Autodesk Fusion 360 part; units mm, degrees
(part 2 of 2)
sketch "Sketch12" plane through (3, 0, 0) normal (1, 0, 0) x (0, 1, 0)
  line L0 (29.3, 0) -> (29.3, 33.5)
  line L1 (29.3, 33.5) -> (-3, 33.5)
  line L2 (-3, 33.5) -> (-3, 0)
  line L3 (-3, 0) -> (29.3, 0)
  spline S0 degree 3 poles (16.8231, 27.7956) (16.7769, 27.7883) (16.6969, 27.7776) (16.6456, 27.7708) knots 0 0 0 0 1 1 1 1
  spline S1 degree 3 poles (16.6456, 27.7708) (16.5335, 27.7568) (16.4265, 27.7404) (16.347, 27.7252) knots 0 0 0 0 1 1 1 1
  spline S2 degree 3 poles (16.347, 27.7252) (16.2124, 27.6987) (15.9471, 27.6266) (15.8192, 27.5815) knots 0 0 0 0 1 1 1 1
  spline S3 degree 3 poles (15.8192, 27.5815) (15.7702, 27.5641) (15.7088, 27.5427) (15.6823, 27.5331) knots 0 0 0 0 1 1 1 1
  spline S4 degree 3 poles (15.6823, 27.5331) (15.6558, 27.5241) (15.6271, 27.5134) (15.6175, 27.5089) knots 0 0 0 0 1 1 1 1
  spline S5 degree 3 poles (15.6175, 27.5089) (15.6085, 27.5049) (15.569, 27.4886) (15.5302, 27.4723) knots 0 0 0 0 1 1 1 1
  spline S6 degree 3 poles (15.5302, 27.4723) (15.4913, 27.4559) (15.4575, 27.4413) (15.4541, 27.4385) knots 0 0 0 0 1 1 1 1
  spline S7 degree 3 poles (15.4541, 27.4385) (15.4513, 27.4362) (15.4231, 27.4238) (15.3921, 27.4108) knots 0 0 0 0 1 1 1 1
  spline S8 degree 3 poles (15.3921, 27.4108) (15.3612, 27.3973) (15.3093, 27.3725) (15.2767, 27.3556) knots 0 0 0 0 1 1 1 1
  spline S9 degree 3 poles (15.2767, 27.3556) (15.244, 27.3382) (15.1888, 27.3094) (15.1544, 27.2914) knots 0 0 0 0 1 1 1 1
  spline S10 degree 3 poles (15.1544, 27.2914) (15.0609, 27.2435) (14.8051, 27.0869) (14.7499, 27.0447) knots 0 0 0 0 1 1 1 1
  spline S11 degree 3 poles (14.7499, 27.0447) (14.7375, 27.0351) (14.7082, 27.0142) (14.6851, 26.9979) knots 0 0 0 0 1 1 1 1
  spline S12 degree 3 poles (14.6851, 26.9979) (14.5792, 26.9247) (14.4277, 26.8069) (14.3105, 26.7066) knots 0 0 0 0 1 1 1 1
  spline S13 degree 3 poles (14.3105, 26.7066) (14.217, 26.6272) (14.1561, 26.5692) (14.0175, 26.43) knots 0 0 0 0 1 1 1 1
  spline S14 degree 3 poles (14.0175, 26.43) (13.8209, 26.2323) (13.817, 26.2283) (13.7522, 26.154) knots 0 0 0 0 1 1 1 1
  spline S15 degree 3 poles (13.7522, 26.154) (13.6406, 26.0272) (13.5837, 25.9562) (13.4299, 25.754) knots 0 0 0 0 1 1 1 1
  spline S16 degree 3 poles (13.4299, 25.754) (13.3916, 25.7038) (13.2761, 25.5326) (13.2006, 25.4148) knots 0 0 0 0 1 1 1 1
  spline S17 degree 3 poles (13.2006, 25.4148) (13.1145, 25.2796) (12.9691, 25.0013) (12.9077, 24.8526) knots 0 0 0 0 1 1 1 1
  spline S18 degree 3 poles (12.9077, 24.8526) (12.893, 24.8171) (12.875, 24.7754) (12.8683, 24.7596) knots 0 0 0 0 1 1 1 1
  spline S19 degree 3 poles (12.8683, 24.7596) (12.8491, 24.7157) (12.8316, 24.6706) (12.8294, 24.6571) knots 0 0 0 0 1 1 1 1
  spline S20 degree 3 poles (12.8294, 24.6571) (12.8277, 24.6503) (12.8153, 24.6137) (12.8018, 24.5754) knots 0 0 0 0 1 1 1 1
  spline S21 degree 3 poles (12.8018, 24.5754) (12.7809, 24.5168) (12.7623, 24.4611) (12.7297, 24.354) knots 0 0 0 0 1 1 1 1
  spline S22 degree 3 poles (12.7297, 24.354) (12.7269, 24.345) (12.7235, 24.3298) (12.7223, 24.3202) knots 0 0 0 0 1 1 1 1
  spline S23 degree 3 poles (12.7223, 24.3202) (12.7212, 24.3112) (12.71, 24.2616) (12.697, 24.2104) knots 0 0 0 0 1 1 1 1
  spline S24 degree 3 poles (12.697, 24.2104) (12.6514, 24.0239) (12.6215, 23.8419) (12.6147, 23.7061) knots 0 0 0 0 1 1 1 1
  spline S25 degree 3 poles (12.6147, 23.7061) (12.6136, 23.6785) (12.6097, 23.6177) (12.6069, 23.5709) knots 0 0 0 0 1 1 1 1
  spline S26 degree 3 poles (12.6069, 23.5709) (12.5995, 23.4645) (12.5995, 23.3062) (12.6063, 23.2076) knots 0 0 0 0 1 1 1 1
  spline S27 degree 3 poles (12.6063, 23.2076) (12.6097, 23.1659) (12.6131, 23.105) (12.6147, 23.0724) knots 0 0 0 0 1 1 1 1
  spline S28 degree 3 poles (12.6147, 23.0724) (12.6164, 23.0397) (12.6232, 22.9602) (12.63, 22.8955) knots 0 0 0 0 1 1 1 1
  line L4 (12.63, 22.8955) -> (12.6418, 22.7777)
  line L5 (12.6418, 22.7777) -> (12.7466, 22.7817)
  spline S29 degree 3 poles (12.7466, 22.7817) (12.9922, 22.7907) (13.2373, 22.8177) (13.4654, 22.8617) knots 0 0 0 0 1 1 1 1
  spline S30 degree 3 poles (13.4654, 22.8617) (13.6063, 22.8887) (13.8863, 22.9698) (14.0271, 23.0245) knots 0 0 0 0 1 1 1 1
  spline S31 degree 3 poles (14.0271, 23.0245) (14.0879, 23.0476) (14.1392, 23.0667) (14.1415, 23.0667) knots 0 0 0 0 1 1 1 1
  spline S32 degree 3 poles (14.1415, 23.0667) (14.1437, 23.0667) (14.1589, 23.0729) (14.1747, 23.0802) knots 0 0 0 0 1 1 1 1
  spline S33 degree 3 poles (14.1747, 23.0802) (14.1905, 23.0876) (14.2277, 23.1045) (14.257, 23.1174) knots 0 0 0 0 1 1 1 1
  spline S34 degree 3 poles (14.257, 23.1174) (14.3122, 23.1417) (14.3206, 23.1456) (14.4485, 23.2104) knots 0 0 0 0 1 1 1 1
  spline S35 degree 3 poles (14.4485, 23.2104) (14.5662, 23.2695) (14.8367, 23.4278) (14.8485, 23.4442) knots 0 0 0 0 1 1 1 1
  spline S36 degree 3 poles (14.8485, 23.4442) (14.8502, 23.4464) (14.8795, 23.4673) (14.9133, 23.4904) knots 0 0 0 0 1 1 1 1
  spline S37 degree 3 poles (14.9133, 23.4904) (14.9967, 23.5473) (15.0958, 23.62) (15.1809, 23.6887) knots 0 0 0 0 1 1 1 1
  spline S38 degree 3 poles (15.1809, 23.6887) (15.2474, 23.7422) (15.2676, 23.7597) (15.3747, 23.8571) knots 0 0 0 0 1 1 1 1
  spline S39 degree 3 poles (15.3747, 23.8571) (15.533, 24.0008) (15.7921, 24.2695) (15.911, 24.4132) knots 0 0 0 0 1 1 1 1
  spline S40 degree 3 poles (15.911, 24.4132) (15.9589, 24.4712) (16.0958, 24.652) (16.1414, 24.718) knots 0 0 0 0 1 1 1 1
  spline S41 degree 3 poles (16.1414, 24.718) (16.1572, 24.7405) (16.173, 24.7619) (16.1769, 24.7658) knots 0 0 0 0 1 1 1 1
  spline S42 degree 3 poles (16.1769, 24.7658) (16.1876, 24.7771) (16.3093, 24.9698) (16.3335, 25.0137) knots 0 0 0 0 1 1 1 1
  spline S43 degree 3 poles (16.3335, 25.0137) (16.3448, 25.0351) (16.36, 25.0605) (16.3673, 25.0706) knots 0 0 0 0 1 1 1 1
  spline S44 degree 3 poles (16.3673, 25.0706) (16.3825, 25.0909) (16.5386, 25.3895) (16.5386, 25.3979) knots 0 0 0 0 1 1 1 1
  spline S45 degree 3 poles (16.5386, 25.3979) (16.5386, 25.4008) (16.5516, 25.4312) (16.5673, 25.4644) knots 0 0 0 0 1 1 1 1
  spline S46 degree 3 poles (16.5673, 25.4644) (16.6011, 25.5371) (16.6456, 25.6436) (16.649, 25.6605) knots 0 0 0 0 1 1 1 1
  spline S47 degree 3 poles (16.649, 25.6605) (16.6501, 25.6672) (16.6535, 25.6774) (16.6569, 25.6836) knots 0 0 0 0 1 1 1 1
  spline S48 degree 3 poles (16.6569, 25.6836) (16.6761, 25.7213) (16.7448, 25.9224) (16.7504, 25.9568) knots 0 0 0 0 1 1 1 1
  spline S49 degree 3 poles (16.7504, 25.9568) (16.7515, 25.9647) (16.7566, 25.981) (16.7611, 25.9934) knots 0 0 0 0 1 1 1 1
  spline S50 degree 3 poles (16.7611, 25.9934) (16.7752, 26.0329) (16.8361, 26.2706) (16.8484, 26.3331) knots 0 0 0 0 1 1 1 1
  spline S51 degree 3 poles (16.8484, 26.3331) (16.8817, 26.5083) (16.9087, 26.7061) (16.9256, 26.8892) knots 0 0 0 0 1 1 1 1
  spline S52 degree 3 poles (16.9256, 26.8892) (16.942, 27.0728) (16.938, 27.5494) (16.9183, 27.7725) knots 0 0 0 0 1 1 1 1
  spline S53 degree 3 poles (16.9183, 27.7725) (16.916, 27.7934) (16.9132, 27.8097) (16.911, 27.8097) knots 0 0 0 0 1 1 1 1
  spline S54 degree 3 poles (16.911, 27.8097) (16.9093, 27.8091) (16.8699, 27.8029) (16.8231, 27.7956) knots 0 0 0 0 1 1 1 1
  spline S55 degree 3 poles (9.1782, 23.0498) (8.8909, 23.0335) (8.6036, 23.0002) (8.3163, 22.9507) knots 0 0 0 0 1 1 1 1
  spline S56 degree 3 poles (8.3163, 22.9507) (8.1613, 22.9236) (7.8334, 22.8414) (7.674, 22.7901) knots 0 0 0 0 1 1 1 1
  spline S57 degree 3 poles (7.674, 22.7901) (7.5208, 22.7405) (7.4537, 22.718) (7.4318, 22.709) knots 0 0 0 0 1 1 1 1
  spline S58 degree 3 poles (7.4318, 22.709) (7.4228, 22.7045) (7.3591, 22.6797) (7.2915, 22.6526) knots 0 0 0 0 1 1 1 1
  spline S59 degree 3 poles (7.2915, 22.6526) (7.2239, 22.6262) (7.145, 22.5929) (7.1168, 22.5794) knots 0 0 0 0 1 1 1 1
  spline S60 degree 3 poles (7.1168, 22.5794) (7.0887, 22.5659) (7.0329, 22.54) (6.9923, 22.5214) knots 0 0 0 0 1 1 1 1
  spline S61 degree 3 poles (6.9923, 22.5214) (6.9523, 22.5034) (6.8966, 22.4752) (6.8684, 22.4589) knots 0 0 0 0 1 1 1 1
  spline S62 degree 3 poles (6.8684, 22.4589) (6.8408, 22.4431) (6.816, 22.4301) (6.8138, 22.4301) knots 0 0 0 0 1 1 1 1
  spline S63 degree 3 poles (6.8138, 22.4301) (6.7985, 22.4301) (6.469, 22.2335) (6.3783, 22.1698) knots 0 0 0 0 1 1 1 1
  spline S64 degree 3 poles (6.3783, 22.1698) (6.2059, 22.0498) (6.0465, 21.9287) (5.9276, 21.8284) knots 0 0 0 0 1 1 1 1
  spline S65 degree 3 poles (5.9276, 21.8284) (5.7873, 21.7096) (5.4853, 21.4104) (5.3608, 21.2662) knots 0 0 0 0 1 1 1 1
  spline S66 degree 3 poles (5.3608, 21.2662) (5.2566, 21.1462) (5.1738, 21.042) (5.0769, 20.909) knots 0 0 0 0 1 1 1 1
  spline S67 degree 3 poles (5.0769, 20.909) (5.0459, 20.8673) (5.0177, 20.8296) (5.0138, 20.8257) knots 0 0 0 0 1 1 1 1
  spline S68 degree 3 poles (5.0138, 20.8257) (5.0037, 20.8155) (4.8876, 20.6397) (4.8454, 20.571) knots 0 0 0 0 1 1 1 1
  spline S69 degree 3 poles (4.8454, 20.571) (4.8273, 20.5417) (4.811, 20.5164) (4.8093, 20.5147) knots 0 0 0 0 1 1 1 1
  spline S70 degree 3 poles (4.8093, 20.5147) (4.7941, 20.5028) (4.6409, 20.224) (4.5687, 20.0775) knots 0 0 0 0 1 1 1 1
  spline S71 degree 3 poles (4.5687, 20.0775) (4.4865, 19.9113) (4.46, 19.8538) (4.4149, 19.7457) knots 0 0 0 0 1 1 1 1
  spline S72 degree 3 poles (4.4149, 19.7457) (4.3547, 19.6009) (4.3406, 19.566) (4.3383, 19.5541) knots 0 0 0 0 1 1 1 1
  spline S73 degree 3 poles (4.3383, 19.5541) (4.3372, 19.5479) (4.3299, 19.5265) (4.322, 19.5062) knots 0 0 0 0 1 1 1 1
  spline S74 degree 3 poles (4.322, 19.5062) (4.3006, 19.4539) (4.2403, 19.2854) (4.2386, 19.2753) knots 0 0 0 0 1 1 1 1
  spline S75 degree 3 poles (4.2386, 19.2753) (4.2375, 19.2708) (4.2352, 19.2634) (4.233, 19.2601) knots 0 0 0 0 1 1 1 1
  spline S76 degree 3 poles (4.233, 19.2601) (4.2302, 19.2561) (4.2296, 19.2527) (4.2307, 19.2527) knots 0 0 0 0 1 1 1 1
  spline S77 degree 3 poles (4.2307, 19.2527) (4.2324, 19.2527) (4.2262, 19.2291) (4.2166, 19.2009) knots 0 0 0 0 1 1 1 1
  spline S78 degree 3 poles (4.2166, 19.2009) (4.1755, 19.0708) (4.1366, 18.9384) (4.1316, 18.9091) knots 0 0 0 0 1 1 1 1
  spline S79 degree 3 poles (4.1316, 18.9091) (4.1299, 18.9012) (4.1186, 18.8539) (4.1057, 18.8037) knots 0 0 0 0 1 1 1 1
  spline S80 degree 3 poles (4.1057, 18.8037) (4.0679, 18.6539) (4.0279, 18.4708) (4.0228, 18.428) knots 0 0 0 0 1 1 1 1
  spline S81 degree 3 poles (4.0228, 18.428) (4.0217, 18.4156) (4.0166, 18.384) (4.0121, 18.3575) knots 0 0 0 0 1 1 1 1
  spline S82 degree 3 poles (4.0121, 18.3575) (3.9631, 18.0871) (3.9231, 17.7852) (3.9169, 17.6443) knots 0 0 0 0 1 1 1 1
  spline S83 degree 3 poles (3.9169, 17.6443) (3.9152, 17.6105) (3.9102, 17.5294) (3.9057, 17.464) knots 0 0 0 0 1 1 1 1
  spline S84 degree 3 poles (3.9057, 17.464) (3.8893, 17.2364) (3.8837, 17.0173) (3.8871, 16.7204) knots 0 0 0 0 1 1 1 1
  spline S85 degree 3 poles (3.8871, 16.7204) (3.8904, 16.4393) (3.8938, 16.3463) (3.9107, 16.0951) knots 0 0 0 0 1 1 1 1
  spline S86 degree 3 poles (3.9107, 16.0951) (3.9147, 16.0269) (3.9186, 15.957) (3.9186, 15.9401) knots 0 0 0 0 1 1 1 1
  spline S87 degree 3 poles (3.9186, 15.9401) (3.9192, 15.8522) (3.9721, 15.4027) (4.0093, 15.1655) knots 0 0 0 0 1 1 1 1
  spline S88 degree 3 poles (4.0093, 15.1655) (4.0149, 15.1283) (4.0217, 15.0804) (4.0234, 15.0596) knots 0 0 0 0 1 1 1 1
  spline S89 degree 3 poles (4.0234, 15.0596) (4.0262, 15.0264) (4.0437, 14.9244) (4.0741, 14.7627) knots 0 0 0 0 1 1 1 1
  spline S90 degree 3 poles (4.0741, 14.7627) (4.0792, 14.7362) (4.0933, 14.6669) (4.1057, 14.6078) knots 0 0 0 0 1 1 1 1
  spline S91 degree 3 poles (4.1057, 14.6078) (4.1175, 14.5492) (4.1287, 14.49) (4.1299, 14.4776) knots 0 0 0 0 1 1 1 1
  spline S92 degree 3 poles (4.1299, 14.4776) (4.1327, 14.45) (4.1513, 14.3672) (4.1935, 14.1965) knots 0 0 0 0 1 1 1 1
  spline S93 degree 3 poles (4.1935, 14.1965) (4.2104, 14.1283) (4.2279, 14.0551) (4.2318, 14.0331) knots 0 0 0 0 1 1 1 1
  spline S94 degree 3 poles (4.2318, 14.0331) (4.2425, 13.9791) (4.2831, 13.8275) (4.3299, 13.6686) knots 0 0 0 0 1 1 1 1
  spline S95 degree 3 poles (4.3299, 13.6686) (4.3361, 13.6472) (4.3394, 13.6303) (4.3378, 13.6303) knots 0 0 0 0 1 1 1 1
  spline S96 degree 3 poles (4.3378, 13.6303) (4.3361, 13.6303) (4.3378, 13.627) (4.3411, 13.623) knots 0 0 0 0 1 1 1 1
  spline S97 degree 3 poles (4.3411, 13.623) (4.3445, 13.6185) (4.3462, 13.614) (4.3445, 13.6123) knots 0 0 0 0 1 1 1 1
  spline S98 degree 3 poles (4.3445, 13.6123) (4.3417, 13.6095) (4.3547, 13.5655) (4.4132, 13.3824) knots 0 0 0 0 1 1 1 1
  spline S99 degree 3 poles (4.4132, 13.3824) (4.4307, 13.3284) (4.4454, 13.2788) (4.4465, 13.2726) knots 0 0 0 0 1 1 1 1
  spline S100 degree 3 poles (4.4465, 13.2726) (4.4471, 13.2664) (4.4707, 13.1948) (4.4989, 13.1132) knots 0 0 0 0 1 1 1 1
  spline S101 degree 3 poles (4.4989, 13.1132) (4.5271, 13.0315) (4.5513, 12.9594) (4.5524, 12.9526) knots 0 0 0 0 1 1 1 1
  spline S102 degree 3 poles (4.5524, 12.9526) (4.5552, 12.9402) (4.5992, 12.818) (4.6369, 12.7182) knots 0 0 0 0 1 1 1 1
  spline S103 degree 3 poles (4.6369, 12.7182) (4.6482, 12.6895) (4.6572, 12.663) (4.6572, 12.6596) knots 0 0 0 0 1 1 1 1
  spline S104 degree 3 poles (4.6572, 12.6596) (4.6572, 12.6568) (4.6825, 12.5904) (4.713, 12.5126) knots 0 0 0 0 1 1 1 1
  spline S105 degree 3 poles (4.713, 12.5126) (4.7439, 12.4349) (4.7777, 12.3487) (4.789, 12.3205) knots 0 0 0 0 1 1 1 1
  spline S106 degree 3 poles (4.789, 12.3205) (4.7997, 12.2929) (4.8228, 12.2371) (4.8403, 12.1966) knots 0 0 0 0 1 1 1 1
  spline S107 degree 3 poles (4.8403, 12.1966) (4.8577, 12.1566) (4.873, 12.1188) (4.8741, 12.1137) knots 0 0 0 0 1 1 1 1
  spline S108 degree 3 poles (4.8741, 12.1137) (4.8752, 12.1087) (4.8927, 12.0681) (4.9124, 12.0236) knots 0 0 0 0 1 1 1 1
  spline S109 degree 3 poles (4.9124, 12.0236) (4.9321, 11.9791) (4.967, 11.9014) (4.9896, 11.8501) knots 0 0 0 0 1 1 1 1
  spline S110 degree 3 poles (4.9896, 11.8501) (5.0121, 11.7988) (5.0414, 11.7346) (5.0555, 11.7064) knots 0 0 0 0 1 1 1 1
  spline S111 degree 3 poles (5.0555, 11.7064) (5.0696, 11.6788) (5.082, 11.6512) (5.0831, 11.6456) knots 0 0 0 0 1 1 1 1
  spline S112 degree 3 poles (5.0831, 11.6456) (5.0876, 11.6197) (5.4177, 10.9622) (5.478, 10.8586) knots 0 0 0 0 1 1 1 1
  spline S113 degree 3 poles (5.478, 10.8586) (5.4876, 10.8417) (5.5056, 10.8084) (5.5174, 10.7853) knots 0 0 0 0 1 1 1 1
  spline S114 degree 3 poles (5.5174, 10.7853) (5.558, 10.7087) (5.6222, 10.591) (5.6318, 10.5769) knots 0 0 0 0 1 1 1 1
  spline S115 degree 3 poles (5.6318, 10.5769) (5.6369, 10.569) (5.6611, 10.5273) (5.6853, 10.4839) knots 0 0 0 0 1 1 1 1
  spline S116 degree 3 poles (5.6853, 10.4839) (5.7096, 10.4405) (5.7372, 10.3921) (5.7467, 10.3763) knots 0 0 0 0 1 1 1 1
  spline S117 degree 3 poles (5.7467, 10.3763) (5.7563, 10.36) (5.7783, 10.3234) (5.7958, 10.2946) knots 0 0 0 0 1 1 1 1
  spline S118 degree 3 poles (5.7958, 10.2946) (5.8132, 10.2653) (5.838, 10.2225) (5.8515, 10.1994) knots 0 0 0 0 1 1 1 1
  spline S119 degree 3 poles (5.8515, 10.1994) (5.865, 10.1763) (5.8881, 10.1386) (5.9034, 10.116) knots 0 0 0 0 1 1 1 1
  spline S120 degree 3 poles (5.9034, 10.116) (5.918, 10.0935) (5.9304, 10.0744) (5.9304, 10.0727) knots 0 0 0 0 1 1 1 1
  spline S121 degree 3 poles (5.9304, 10.0727) (5.9304, 10.0715) (5.9546, 10.0315) (5.9839, 9.9848) knots 0 0 0 0 1 1 1 1
  spline S122 degree 3 poles (5.9839, 9.9848) (6.0132, 9.938) (6.0374, 9.8986) (6.0374, 9.8975) knots 0 0 0 0 1 1 1 1
  spline S123 degree 3 poles (6.0374, 9.8975) (6.0374, 9.8958) (6.0797, 9.8315) (6.1129, 9.7825) knots 0 0 0 0 1 1 1 1
  spline S124 degree 3 poles (6.1129, 9.7825) (6.1203, 9.7718) (6.1597, 9.711) (6.2014, 9.6473) knots 0 0 0 0 1 1 1 1
  spline S125 degree 3 poles (6.2014, 9.6473) (6.2425, 9.5837) (6.2938, 9.5076) (6.3152, 9.4783) knots 0 0 0 0 1 1 1 1
  spline S126 degree 3 poles (6.3152, 9.4783) (6.336, 9.449) (6.3884, 9.3752) (6.4312, 9.3149) knots 0 0 0 0 1 1 1 1
  spline S127 degree 3 poles (6.4312, 9.3149) (6.5095, 9.2034) (6.5811, 9.1071) (6.6374, 9.0361) knots 0 0 0 0 1 1 1 1
  spline S128 degree 3 poles (6.6374, 9.0361) (6.6549, 9.0147) (6.6949, 8.964) (6.7264, 8.9234) knots 0 0 0 0 1 1 1 1
  spline S129 degree 3 poles (6.7264, 8.9234) (6.8307, 8.7899) (6.9907, 8.5995) (7.0599, 8.5262) knots 0 0 0 0 1 1 1 1
  spline S130 degree 3 poles (7.0599, 8.5262) (7.3157, 8.2569) (7.4656, 8.111) (7.6137, 7.9865) knots 0 0 0 0 1 1 1 1
  spline S131 degree 3 poles (7.6137, 7.9865) (7.8205, 7.813) (8.0357, 7.6603) (8.2194, 7.5567) knots 0 0 0 0 1 1 1 1
  spline S132 degree 3 poles (8.2194, 7.5567) (8.2436, 7.5432) (8.2802, 7.5223) (8.301, 7.5105) knots 0 0 0 0 1 1 1 1
  spline S133 degree 3 poles (8.301, 7.5105) (8.3219, 7.4981) (8.3692, 7.4744) (8.4064, 7.4575) knots 0 0 0 0 1 1 1 1
  spline S134 degree 3 poles (8.4064, 7.4575) (8.4436, 7.4406) (8.4768, 7.4243) (8.4796, 7.4215) knots 0 0 0 0 1 1 1 1
  spline S135 degree 3 poles (8.4796, 7.4215) (8.4892, 7.4141) (8.5771, 7.377) (8.6148, 7.3646) knots 0 0 0 0 1 1 1 1
  spline S136 degree 3 poles (8.6148, 7.3646) (8.6334, 7.3584) (8.6565, 7.3499) (8.6655, 7.3454) knots 0 0 0 0 1 1 1 1
  spline S137 degree 3 poles (8.6655, 7.3454) (8.7129, 7.324) (8.8903, 7.2671) (8.9371, 7.2587) knots 0 0 0 0 1 1 1 1
  spline S138 degree 3 poles (8.9371, 7.2587) (8.9517, 7.2564) (8.9991, 7.2463) (9.0413, 7.2372) knots 0 0 0 0 1 1 1 1
  spline S139 degree 3 poles (9.0413, 7.2372) (9.319, 7.1753) (9.6148, 7.1691) (9.9585, 7.217) knots 0 0 0 0 1 1 1 1
  spline S140 degree 3 poles (9.9585, 7.217) (10.0396, 7.2282) (10.19, 7.2558) (10.2683, 7.2733) knots 0 0 0 0 1 1 1 1
  spline S141 degree 3 poles (10.2683, 7.2733) (10.3641, 7.2953) (10.6351, 7.3786) (10.6897, 7.4029) knots 0 0 0 0 1 1 1 1
  spline S142 degree 3 poles (10.6897, 7.4029) (10.7072, 7.4108) (10.7928, 7.4463) (10.8796, 7.4823) knots 0 0 0 0 1 1 1 1
  spline S143 degree 3 poles (10.8796, 7.4823) (10.9663, 7.5178) (11.0401, 7.5488) (11.043, 7.551) knots 0 0 0 0 1 1 1 1
  spline S144 degree 3 poles (11.043, 7.551) (11.0463, 7.5533) (11.0638, 7.5612) (11.0824, 7.5679) knots 0 0 0 0 1 1 1 1
  spline S145 degree 3 poles (11.0824, 7.5679) (11.101, 7.5753) (11.1477, 7.5939) (11.1866, 7.6091) knots 0 0 0 0 1 1 1 1
  spline S146 degree 3 poles (11.1866, 7.6091) (11.2255, 7.6248) (11.3105, 7.6558) (11.3753, 7.6784) knots 0 0 0 0 1 1 1 1
  spline S147 degree 3 poles (11.3753, 7.6784) (11.4407, 7.7009) (11.5117, 7.7262) (11.5331, 7.7341) knots 0 0 0 0 1 1 1 1
  spline S148 degree 3 poles (11.5331, 7.7341) (11.6007, 7.76) (11.6841, 7.7893) (11.7105, 7.7967) knots 0 0 0 0 1 1 1 1
  spline S149 degree 3 poles (11.7105, 7.7967) (11.7246, 7.8006) (11.7872, 7.8203) (11.8497, 7.8406) knots 0 0 0 0 1 1 1 1
  spline S150 degree 3 poles (11.8497, 7.8406) (11.9719, 7.8806) (12.3026, 7.9646) (12.426, 7.9876) knots 0 0 0 0 1 1 1 1
  spline S151 degree 3 poles (12.426, 7.9876) (12.5026, 8.0017) (12.7184, 8.031) (12.8232, 8.0417) knots 0 0 0 0 1 1 1 1
  spline S152 degree 3 poles (12.8232, 8.0417) (13.0784, 8.0676) (13.4418, 8.0564) (13.7499, 8.0136) knots 0 0 0 0 1 1 1 1
  spline S153 degree 3 poles (13.7499, 8.0136) (13.7916, 8.0079) (13.8401, 8.0017) (13.857, 7.9995) knots 0 0 0 0 1 1 1 1
  spline S154 degree 3 poles (13.857, 7.9995) (13.9088, 7.9938) (14.0857, 7.9527) (14.1753, 7.9262) knots 0 0 0 0 1 1 1 1
  spline S155 degree 3 poles (14.1753, 7.9262) (14.222, 7.9122) (14.2727, 7.8969) (14.2891, 7.8924) knots 0 0 0 0 1 1 1 1
  spline S156 degree 3 poles (14.2891, 7.8924) (14.3054, 7.8879) (14.3612, 7.8677) (14.413, 7.8468) knots 0 0 0 0 1 1 1 1
  spline S157 degree 3 poles (14.413, 7.8468) (14.4648, 7.8265) (14.5257, 7.804) (14.5471, 7.7967) knots 0 0 0 0 1 1 1 1
  spline S158 degree 3 poles (14.5471, 7.7967) (14.5691, 7.7893) (14.626, 7.7679) (14.6738, 7.7488) knots 0 0 0 0 1 1 1 1
  spline S159 degree 3 poles (14.6738, 7.7488) (14.7217, 7.7302) (14.7792, 7.7082) (14.8006, 7.7003) knots 0 0 0 0 1 1 1 1
  spline S160 degree 3 poles (14.8006, 7.7003) (14.8913, 7.6671) (14.92, 7.6564) (14.9443, 7.6457) knots 0 0 0 0 1 1 1 1
  spline S161 degree 3 poles (14.9443, 7.6457) (14.9809, 7.6293) (15.2682, 7.5212) (15.3443, 7.4947) knots 0 0 0 0 1 1 1 1
  spline S162 degree 3 poles (15.3443, 7.4947) (15.5043, 7.4401) (15.6276, 7.3989) (15.6795, 7.3837) knots 0 0 0 0 1 1 1 1
  spline S163 degree 3 poles (15.6795, 7.3837) (16.0118, 7.2846) (16.2676, 7.2288) (16.5442, 7.1956) knots 0 0 0 0 1 1 1 1
  spline S164 degree 3 poles (16.5442, 7.1956) (16.6349, 7.1843) (16.8907, 7.1865) (16.9775, 7.1984) knots 0 0 0 0 1 1 1 1
  spline S165 degree 3 poles (16.9775, 7.1984) (17.1634, 7.2249) (17.3651, 7.2789) (17.5115, 7.3409) knots 0 0 0 0 1 1 1 1
  spline S166 degree 3 poles (17.5115, 7.3409) (17.5436, 7.3544) (17.5729, 7.3657) (17.5769, 7.3657) knots 0 0 0 0 1 1 1 1
  spline S167 degree 3 poles (17.5769, 7.3657) (17.5848, 7.3657) (17.8405, 7.493) (17.8879, 7.5206) knots 0 0 0 0 1 1 1 1
  spline S168 degree 3 poles (17.8879, 7.5206) (17.9036, 7.5296) (17.9301, 7.5465) (17.9476, 7.5584) knots 0 0 0 0 1 1 1 1
  spline S169 degree 3 poles (17.9476, 7.5584) (17.965, 7.5702) (17.9814, 7.5798) (17.9831, 7.5798) knots 0 0 0 0 1 1 1 1
  spline S170 degree 3 poles (17.9831, 7.5798) (17.9898, 7.5798) (18.1538, 7.6862) (18.205, 7.7234) knots 0 0 0 0 1 1 1 1
  spline S171 degree 3 poles (18.205, 7.7234) (18.2991, 7.7916) (18.3115, 7.8012) (18.3746, 7.8491) knots 0 0 0 0 1 1 1 1
  spline S172 degree 3 poles (18.3746, 7.8491) (18.7661, 8.1482) (19.1706, 8.5471) (19.5813, 9.0389) knots 0 0 0 0 1 1 1 1
  spline S173 degree 3 poles (19.5813, 9.0389) (19.7892, 9.2885) (19.9058, 9.4372) (20.0416, 9.6259) knots 0 0 0 0 1 1 1 1
  spline S174 degree 3 poles (20.0416, 9.6259) (20.0698, 9.6648) (20.0979, 9.7031) (20.1047, 9.7104) knots 0 0 0 0 1 1 1 1
  spline S175 degree 3 poles (20.1047, 9.7104) (20.1182, 9.7268) (20.1492, 9.7707) (20.2427, 9.9093) knots 0 0 0 0 1 1 1 1
  spline S176 degree 3 poles (20.2427, 9.9093) (20.2805, 9.9651) (20.3216, 10.0248) (20.3346, 10.0417) knots 0 0 0 0 1 1 1 1
  spline S177 degree 3 poles (20.3346, 10.0417) (20.3475, 10.0586) (20.3582, 10.0744) (20.3582, 10.0766) knots 0 0 0 0 1 1 1 1
  spline S178 degree 3 poles (20.3582, 10.0766) (20.3582, 10.0789) (20.3819, 10.1166) (20.4106, 10.1611) knots 0 0 0 0 1 1 1 1
  spline S179 degree 3 poles (20.4106, 10.1611) (20.4399, 10.2056) (20.4647, 10.2445) (20.4658, 10.2484) knots 0 0 0 0 1 1 1 1
  spline S180 degree 3 poles (20.4658, 10.2484) (20.467, 10.2518) (20.4889, 10.2873) (20.5148, 10.3273) knots 0 0 0 0 1 1 1 1
  spline S181 degree 3 poles (20.5148, 10.3273) (20.5627, 10.4005) (20.6726, 10.5842) (20.6782, 10.5994) knots 0 0 0 0 1 1 1 1
  spline S182 degree 3 poles (20.6782, 10.5994) (20.6799, 10.6039) (20.6867, 10.6158) (20.6934, 10.6248) knots 0 0 0 0 1 1 1 1
  spline S183 degree 3 poles (20.6934, 10.6248) (20.7092, 10.6467) (20.7509, 10.72) (20.7869, 10.7893) knots 0 0 0 0 1 1 1 1
  spline S184 degree 3 poles (20.7869, 10.7893) (20.8033, 10.8197) (20.8213, 10.8518) (20.8275, 10.8603) knots 0 0 0 0 1 1 1 1
  spline S185 degree 3 poles (20.8275, 10.8603) (20.8602, 10.9076) (21.2061, 11.5943) (21.2117, 11.6242) knots 0 0 0 0 1 1 1 1
  spline S186 degree 3 poles (21.2117, 11.6242) (21.2128, 11.6293) (21.223, 11.6523) (21.2343, 11.6754) knots 0 0 0 0 1 1 1 1
  spline S187 degree 3 poles (21.2343, 11.6754) (21.2641, 11.7363) (21.3041, 11.8259) (21.3159, 11.8585) knots 0 0 0 0 1 1 1 1
  spline S188 degree 3 poles (21.3159, 11.8585) (21.3255, 11.8839) (21.3458, 11.9307) (21.401, 12.054) knots 0 0 0 0 1 1 1 1
  spline S189 degree 3 poles (21.401, 12.054) (21.41, 12.0743) (21.419, 12.0963) (21.4202, 12.1019) knots 0 0 0 0 1 1 1 1
  spline S190 degree 3 poles (21.4202, 12.1019) (21.4213, 12.1076) (21.4354, 12.1436) (21.4512, 12.1825) knots 0 0 0 0 1 1 1 1
  spline S191 degree 3 poles (21.4512, 12.1825) (21.5002, 12.3008) (21.5289, 12.374) (21.5266, 12.374) knots 0 0 0 0 1 1 1 1
  spline S192 degree 3 poles (21.5266, 12.374) (21.5244, 12.374) (21.543, 12.4247) (21.5526, 12.4444) knots 0 0 0 0 1 1 1 1
  spline S193 degree 3 poles (21.5526, 12.4444) (21.5559, 12.4506) (21.5689, 12.4839) (21.5813, 12.5177) knots 0 0 0 0 1 1 1 1
  spline S194 degree 3 poles (21.5813, 12.5177) (21.5942, 12.552) (21.6117, 12.5982) (21.6202, 12.6208) knots 0 0 0 0 1 1 1 1
  spline S195 degree 3 poles (21.6202, 12.6208) (21.6292, 12.6427) (21.6348, 12.6613) (21.6337, 12.6613) knots 0 0 0 0 1 1 1 1
  spline S196 degree 3 poles (21.6337, 12.6613) (21.6326, 12.6613) (21.6393, 12.6833) (21.6489, 12.7098) knots 0 0 0 0 1 1 1 1
  spline S197 degree 3 poles (21.6489, 12.7098) (21.6585, 12.7363) (21.6652, 12.7594) (21.6641, 12.7599) knots 0 0 0 0 1 1 1 1
  spline S198 degree 3 poles (21.6641, 12.7599) (21.663, 12.7611) (21.6455, 12.7695) (21.6252, 12.7785) knots 0 0 0 0 1 1 1 1
  spline S199 degree 3 poles (21.6252, 12.7785) (21.605, 12.7875) (21.5548, 12.8146) (21.5142, 12.8382) knots 0 0 0 0 1 1 1 1
  spline S200 degree 3 poles (21.5142, 12.8382) (21.4731, 12.8619) (21.4382, 12.8811) (21.4359, 12.8811) knots 0 0 0 0 1 1 1 1
  spline S201 degree 3 poles (21.4359, 12.8811) (21.4309, 12.8811) (21.3345, 12.9363) (21.2923, 12.9639) knots 0 0 0 0 1 1 1 1
  spline S202 degree 3 poles (21.2923, 12.9639) (21.2714, 12.9774) (21.2534, 12.9881) (21.2512, 12.9881) knots 0 0 0 0 1 1 1 1
  spline S203 degree 3 poles (21.2512, 12.9881) (21.2438, 12.9881) (21.0607, 13.1036) (20.9447, 13.1808) knots 0 0 0 0 1 1 1 1
  spline S204 degree 3 poles (20.9447, 13.1808) (20.7819, 13.2901) (20.7188, 13.3346) (20.6399, 13.3965) knots 0 0 0 0 1 1 1 1
  spline S205 degree 3 poles (20.6399, 13.3965) (20.6202, 13.4123) (20.5746, 13.4472) (20.5391, 13.4754) knots 0 0 0 0 1 1 1 1
  spline S206 degree 3 poles (20.5391, 13.4754) (20.3199, 13.645) (20.0692, 13.8765) (19.8929, 14.0726) knots 0 0 0 0 1 1 1 1
  spline S207 degree 3 poles (19.8929, 14.0726) (19.716, 14.2698) (19.5211, 14.5312) (19.3971, 14.7368) knots 0 0 0 0 1 1 1 1
  spline S208 degree 3 poles (19.3971, 14.7368) (19.3791, 14.7672) (19.3566, 14.8038) (19.3475, 14.8185) knots 0 0 0 0 1 1 1 1
  spline S209 degree 3 poles (19.3475, 14.8185) (19.3385, 14.8326) (19.3188, 14.8686) (19.3036, 14.8979) knots 0 0 0 0 1 1 1 1
  spline S210 degree 3 poles (19.3036, 14.8979) (19.2878, 14.9272) (19.2591, 14.9818) (19.2399, 15.019) knots 0 0 0 0 1 1 1 1
  spline S211 degree 3 poles (19.2399, 15.019) (19.2202, 15.0562) (19.1949, 15.108) (19.1836, 15.134) knots 0 0 0 0 1 1 1 1
  spline S212 degree 3 poles (19.1836, 15.134) (19.1723, 15.1604) (19.1571, 15.1948) (19.1492, 15.21) knots 0 0 0 0 1 1 1 1
  spline S213 degree 3 poles (19.1492, 15.21) (19.1301, 15.2478) (19.0935, 15.3362) (19.0884, 15.3565) knots 0 0 0 0 1 1 1 1
  spline S214 degree 3 poles (19.0884, 15.3565) (19.0861, 15.3649) (19.0794, 15.383) (19.0737, 15.3959) knots 0 0 0 0 1 1 1 1
  spline S215 degree 3 poles (19.0737, 15.3959) (19.0506, 15.4444) (18.9859, 15.6263) (18.9814, 15.6545) knots 0 0 0 0 1 1 1 1
  spline S216 degree 3 poles (18.9814, 15.6545) (18.9797, 15.6641) (18.9735, 15.6877) (18.9673, 15.7063) knots 0 0 0 0 1 1 1 1
  spline S217 degree 3 poles (18.9673, 15.7063) (18.934, 15.8077) (18.8788, 16.0246) (18.8743, 16.0708) knots 0 0 0 0 1 1 1 1
  spline S218 degree 3 poles (18.8743, 16.0708) (18.8732, 16.0872) (18.8687, 16.1137) (18.8653, 16.1289) knots 0 0 0 0 1 1 1 1
  spline S219 degree 3 poles (18.8653, 16.1289) (18.8546, 16.1751) (18.8332, 16.3035) (18.8208, 16.3908) knots 0 0 0 0 1 1 1 1
  spline S220 degree 3 poles (18.8208, 16.3908) (18.7521, 16.886) (18.765, 17.4088) (18.8568, 17.855) knots 0 0 0 0 1 1 1 1
  spline S221 degree 3 poles (18.8568, 17.855) (18.8676, 17.9063) (18.8749, 17.9497) (18.8732, 17.9519) knots 0 0 0 0 1 1 1 1
  spline S222 degree 3 poles (18.8732, 17.9519) (18.8721, 17.9542) (18.8732, 17.9576) (18.8766, 17.9598) knots 0 0 0 0 1 1 1 1
  spline S223 degree 3 poles (18.8766, 17.9598) (18.8799, 17.9621) (18.8811, 17.9654) (18.8794, 17.9683) knots 0 0 0 0 1 1 1 1
  spline S224 degree 3 poles (18.8794, 17.9683) (18.8754, 17.9745) (18.9149, 18.1266) (18.9509, 18.2443) knots 0 0 0 0 1 1 1 1
  spline S225 degree 3 poles (18.9509, 18.2443) (18.9661, 18.2956) (18.9802, 18.3429) (18.9814, 18.3497) knots 0 0 0 0 1 1 1 1
  spline S226 degree 3 poles (18.9814, 18.3497) (18.9847, 18.3677) (19.0253, 18.4787) (19.0574, 18.5598) knots 0 0 0 0 1 1 1 1
  spline S227 degree 3 poles (19.0574, 18.5598) (19.0732, 18.5987) (19.0867, 18.6347) (19.0878, 18.6398) knots 0 0 0 0 1 1 1 1
  spline S228 degree 3 poles (19.0878, 18.6398) (19.094, 18.6691) (19.2366, 18.9671) (19.3042, 19.091) knots 0 0 0 0 1 1 1 1
  spline S229 degree 3 poles (19.3042, 19.091) (19.356, 19.1863) (19.4309, 19.3074) (19.5216, 19.442) knots 0 0 0 0 1 1 1 1
  spline S230 degree 3 poles (19.5216, 19.442) (19.6067, 19.5682) (19.7194, 19.7186) (19.7949, 19.8076) knots 0 0 0 0 1 1 1 1
  spline S231 degree 3 poles (19.7949, 19.8076) (20.0258, 20.0792) (20.1729, 20.2324) (20.3948, 20.4335) knots 0 0 0 0 1 1 1 1
  spline S232 degree 3 poles (20.3948, 20.4335) (20.4506, 20.4843) (20.5853, 20.6003) (20.6343, 20.6397) knots 0 0 0 0 1 1 1 1
  spline S233 degree 3 poles (20.6343, 20.6397) (20.6484, 20.651) (20.6698, 20.669) (20.6816, 20.6809) knots 0 0 0 0 1 1 1 1
  spline S234 degree 3 poles (20.6816, 20.6809) (20.7227, 20.7186) (20.9402, 20.8831) (21.0602, 20.9671) knots 0 0 0 0 1 1 1 1
  spline S235 degree 3 poles (21.0602, 20.9671) (21.1188, 21.0082) (21.1227, 21.0121) (21.1114, 21.029) knots 0 0 0 0 1 1 1 1
  spline S236 degree 3 poles (21.1114, 21.029) (21.0985, 21.0493) (20.9937, 21.1755) (20.9193, 21.2611) knots 0 0 0 0 1 1 1 1
  spline S237 degree 3 poles (20.9193, 21.2611) (20.6703, 21.5468) (20.3684, 21.8273) (20.0906, 22.0296) knots 0 0 0 0 1 1 1 1
  spline S238 degree 3 poles (20.0906, 22.0296) (20.0596, 22.0521) (20.0315, 22.0741) (20.0281, 22.0786) knots 0 0 0 0 1 1 1 1
  spline S239 degree 3 poles (20.0281, 22.0786) (20.023, 22.0848) (19.8844, 22.1783) (19.7436, 22.2707) knots 0 0 0 0 1 1 1 1
  spline S240 degree 3 poles (19.7436, 22.2707) (19.7109, 22.2915) (19.5109, 22.4076) (19.4619, 22.4335) knots 0 0 0 0 1 1 1 1
  spline S241 degree 3 poles (19.4619, 22.4335) (19.4073, 22.4628) (19.1611, 22.5834) (19.1188, 22.6014) knots 0 0 0 0 1 1 1 1
  spline S242 degree 3 poles (19.1188, 22.6014) (19.0923, 22.6132) (19.0608, 22.6273) (19.0484, 22.6324) knots 0 0 0 0 1 1 1 1
  spline S243 degree 3 poles (19.0484, 22.6324) (19.0152, 22.6476) (18.7994, 22.7315) (18.7667, 22.7422) knots 0 0 0 0 1 1 1 1
  spline S244 degree 3 poles (18.7667, 22.7422) (18.7515, 22.7473) (18.6845, 22.7693) (18.618, 22.7912) knots 0 0 0 0 1 1 1 1
  spline S245 degree 3 poles (18.618, 22.7912) (18.4202, 22.856) (18.08, 22.9388) (17.9019, 22.9653) knots 0 0 0 0 1 1 1 1
  spline S246 degree 3 poles (17.9019, 22.9653) (17.8788, 22.9687) (17.8219, 22.9777) (17.7752, 22.985) knots 0 0 0 0 1 1 1 1
  spline S247 degree 3 poles (17.7752, 22.985) (17.618, 23.0098) (17.4625, 23.0273) (17.2428, 23.0448) knots 0 0 0 0 1 1 1 1
  spline S248 degree 3 poles (17.2428, 23.0448) (17.1211, 23.0543) (16.6704, 23.0577) (16.5239, 23.0504) knots 0 0 0 0 1 1 1 1
  spline S249 degree 3 poles (16.5239, 23.0504) (16.2203, 23.0352) (15.9003, 22.998) (15.6119, 22.945) knots 0 0 0 0 1 1 1 1
  spline S250 degree 3 poles (15.6119, 22.945) (15.4502, 22.9157) (15.1555, 22.8419) (15.0034, 22.7935) knots 0 0 0 0 1 1 1 1
  spline S251 degree 3 poles (15.0034, 22.7935) (14.9386, 22.7726) (14.8778, 22.7535) (14.8682, 22.7512) knots 0 0 0 0 1 1 1 1
  spline S252 degree 3 poles (14.8682, 22.7512) (14.8417, 22.7439) (14.7792, 22.7214) (14.6936, 22.6881) knots 0 0 0 0 1 1 1 1
  spline S253 degree 3 poles (14.6936, 22.6881) (14.6502, 22.6707) (14.5984, 22.651) (14.5781, 22.6442) knots 0 0 0 0 1 1 1 1
  spline S254 degree 3 poles (14.5781, 22.6442) (14.5578, 22.6374) (14.4947, 22.6132) (14.4372, 22.5907) knots 0 0 0 0 1 1 1 1
  spline S255 degree 3 poles (14.4372, 22.5907) (14.3798, 22.5681) (14.3229, 22.5467) (14.3105, 22.5428) knots 0 0 0 0 1 1 1 1
  spline S256 degree 3 poles (14.3105, 22.5428) (14.2981, 22.5388) (14.2525, 22.5214) (14.2091, 22.505) knots 0 0 0 0 1 1 1 1
  spline S257 degree 3 poles (14.2091, 22.505) (14.1657, 22.4881) (14.1048, 22.4645) (14.0739, 22.4527) knots 0 0 0 0 1 1 1 1
  spline S258 degree 3 poles (14.0739, 22.4527) (14.0429, 22.4408) (13.995, 22.4228) (13.9668, 22.4132) knots 0 0 0 0 1 1 1 1
  spline S259 degree 3 poles (13.9668, 22.4132) (13.9392, 22.4031) (13.906, 22.3907) (13.8936, 22.3851) knots 0 0 0 0 1 1 1 1
  spline S260 degree 3 poles (13.8936, 22.3851) (13.7905, 22.3394) (13.4339, 22.2369) (13.3235, 22.2217) knots 0 0 0 0 1 1 1 1
  spline S261 degree 3 poles (13.3235, 22.2217) (13.1854, 22.2031) (13.1544, 22.1991) (13.0857, 22.1929) knots 0 0 0 0 1 1 1 1
  spline S262 degree 3 poles (13.0857, 22.1929) (12.9933, 22.1851) (12.8097, 22.1896) (12.7387, 22.2014) knots 0 0 0 0 1 1 1 1
  spline S263 degree 3 poles (12.7387, 22.2014) (12.7111, 22.2065) (12.6694, 22.2132) (12.6469, 22.216) knots 0 0 0 0 1 1 1 1
  spline S264 degree 3 poles (12.6469, 22.216) (12.5962, 22.2239) (12.4649, 22.2594) (12.364, 22.2932) knots 0 0 0 0 1 1 1 1
  spline S265 degree 3 poles (12.364, 22.2932) (12.3224, 22.3073) (12.2767, 22.322) (12.2626, 22.3259) knots 0 0 0 0 1 1 1 1
  spline S266 degree 3 poles (12.2626, 22.3259) (12.2486, 22.3298) (12.1979, 22.3484) (12.15, 22.3681) knots 0 0 0 0 1 1 1 1
  spline S267 degree 3 poles (12.15, 22.3681) (12.1021, 22.3873) (12.0283, 22.4166) (11.9866, 22.4329) knots 0 0 0 0 1 1 1 1
  spline S268 degree 3 poles (11.9866, 22.4329) (11.9449, 22.4498) (11.8784, 22.4769) (11.8396, 22.4938) knots 0 0 0 0 1 1 1 1
  spline S269 degree 3 poles (11.8396, 22.4938) (11.8001, 22.5112) (11.7562, 22.5293) (11.741, 22.5343) knots 0 0 0 0 1 1 1 1
  spline S270 degree 3 poles (11.741, 22.5343) (11.7258, 22.5394) (11.706, 22.5473) (11.6965, 22.5512) knots 0 0 0 0 1 1 1 1
  spline S271 degree 3 poles (11.6965, 22.5512) (11.6598, 22.5687) (11.5139, 22.629) (11.4767, 22.6425) knots 0 0 0 0 1 1 1 1
  spline S272 degree 3 poles (11.4767, 22.6425) (11.4553, 22.6504) (11.4148, 22.6667) (11.3866, 22.6791) knots 0 0 0 0 1 1 1 1
  spline S273 degree 3 poles (11.3866, 22.6791) (11.3348, 22.7017) (11.2351, 22.7411) (11.1838, 22.7597) knots 0 0 0 0 1 1 1 1
  spline S274 degree 3 poles (11.1838, 22.7597) (11.0897, 22.7935) (10.9139, 22.8526) (10.8852, 22.86) knots 0 0 0 0 1 1 1 1
  spline S275 degree 3 poles (10.8852, 22.86) (10.8666, 22.865) (10.8199, 22.878) (10.781, 22.8893) knots 0 0 0 0 1 1 1 1
  spline S276 degree 3 poles (10.781, 22.8893) (10.6728, 22.9202) (10.532, 22.9541) (10.4813, 22.9602) knots 0 0 0 0 1 1 1 1
  spline S277 degree 3 poles (10.4813, 22.9602) (10.4559, 22.9631) (10.4334, 22.967) (10.4311, 22.9687) knots 0 0 0 0 1 1 1 1
  spline S278 degree 3 poles (10.4311, 22.9687) (10.4232, 22.9732) (10.1956, 23.0098) (10.1021, 23.0211) knots 0 0 0 0 1 1 1 1
  spline S279 degree 3 poles (10.1021, 23.0211) (9.8914, 23.047) (9.8171, 23.051) (9.5359, 23.0526) knots 0 0 0 0 1 1 1 1
  spline S280 degree 3 poles (9.5359, 23.0526) (9.3855, 23.0538) (9.225, 23.0521) (9.1782, 23.0498) knots 0 0 0 0 1 1 1 1
extrude "Extrude23" cut sketch "Sketch12" against normal blind 3 contours S0 S1 S2 S3 S4 S5 S6 S7 S8 S9 S10 S11 S12 S13 S14 S15 S16 S17 S18 S19 S20 S21 S22 S23 S24 S25 S26 S27 S28 L4 L5 S29 S30 S31 S32 S33 S34 S35 S36 S37 S38 S39 S40 S41 S42 S43 S44 S45 S46 S47 S48 S49 S50 S51 S52 S53 S54 | S55 S56 S57 S58 S59 S60 S61 S62 S63 S64 S65 S66 S67 S68 S69 S70 S71 S72 S73 S74 S75 S76 S77 S78 S79 S80 S81 S82 S83 S84 S85 S86 S87 S88 S89 S90 S91 S92 S93 S94 S95 S96 S97 S98 S99 S100 S101 S102 S103 S104 S105 S106 S107 S108 S109 S110 S111 S112 S113 S114 S115 S116 S117 S118 S119 S120 S121 S122 S123 S124 S125 S126 S127 S128 S129 S130 S131 S132 S133 S134 S135 S136 S137 S138 S139 S140 S141 S142 S143 S144 S145 S146 S147 S148 S149 S150 S151 S152 S153 S154 S155 S156 S157 S158 S159 S160 S161 S162 S163 S164 S165 S166 S167 S168 S169 S170 S171 S172 S173 S174 S175 S176 S177 S178 S179 S180 S181 S182 S183 S184 S185 S186 S187 S188 S189 S190 S191 S192 S193 S194 S195 S196 S197 S198 S199 S200 S201 S202 S203 S204 S205 S206 S207 S208 S209 S210 S211 S212 S213 S214 S215 S216 S217 S218 S219 S220 S221 S222 S223 S224 S225 S226 S227 S228 S229 S230 S231 S232 S233 S234 S235 S236 S237 S238 S239 S240 S241 S242 S243 S244 S245 S246 S247 S248 S249 S250 S251 S252 S253 S254 S255 S256 S257 S258 S259 S260 S261 S262 S263 S264 S265 S266 S267 S268 S269 S270 S271 S272 S273 S274 S275 S276 S277 S278 S279 S280 bodies 2
fillet "Fillet6" radius 2 1 edges at (0, 0, 14.25) on bodies 2
fillet "Fillet7" radius 2 1 edges at (0, 26.3, 14.25) on bodies 2
fillet "Fillet8" radius 2 1 edges at (-27, 26.3, 14.25) on bodies 2
fillet "Fillet9" radius 2 1 edges at (-27, 0, 14.25) on bodies 2
fillet "Fillet10" radius 3.5 4 edges at (3, -3, 16.75) (-30, -3, 16.75) (-30, 29.3, 16.75) (3, 29.3, 16.75) on bodies 2
fillet "Fillet11" radius 3.5 4 edges at (-13, 2.5, 33.5) (-2.5, 9.35, 33.5) (-13, 16.2, 33.5) (-23.5, 9.35, 33.5) on bodies 2
fillet "Fillet12" radius 3.5 4 edges at (-13, 2.5, 41.5) (-23.5, 9.35, 41.5) (-13, 16.2, 41.5) (-2.5, 9.35, 41.5) on bodies 2
sketch "Sketch7" plane through (0, 0, 0) normal (0, 0, 1) x (1, 0, 0)
  line L0 (-0.5, 0.5) -> (-26.5, 0.5)
  line L1 (-26.5, 0.5) -> (-26.5, 26)
  line L2 (-26.5, 26) -> (-0.5, 26)
  line L3 (-0.5, 26) -> (-0.5, 0.5)
  constraint horizontal L0
  constraint vertical L1
  constraint horizontal L2
  constraint vertical L3
extrude "Extrude6" add sketch "Sketch7" along normal blind 28 separate body makes body 3
sketch "Sketch8" plane through (0, 0, 28) normal (0, 0, 1) x (-1, 0, 0)
  line L0 (0.5, -26) -> (26.5, -26)
  line L1 (26.5, -26) -> (26.5, -0.5)
  line L2 (26.5, -0.5) -> (0.5, -0.5)
  line L3 (0.5, -0.5) -> (0.5, -26)
  line L4 (19.3023, -11.9206) -> (6.6767, -11.9206)
  line L5 (6.6767, -11.9206) -> (6.6767, -6.6359)
  line L6 (6.6767, -6.6359) -> (19.3023, -6.6359)
  line L7 (19.3023, -6.6359) -> (19.3023, -11.9206)
  constraint horizontal L4
  constraint vertical L5
  constraint horizontal L6
  constraint vertical L7
extrude "Extrude7" add sketch "Sketch8" along normal blind 13.5 contours L4 L5 L6 L7 bodies 3
sketch "Sketch9" plane through (0, 0, 41.5) normal (0, 0, 1) x (-1, 0, 0)
  line L0 (19.3023, -6.6359) -> (6.6767, -6.6359)
  line L1 (6.6767, -6.6359) -> (6.6767, -11.9206)
  line L2 (6.6767, -11.9206) -> (19.3023, -11.9206)
  line L3 (19.3023, -11.9206) -> (19.3023, -6.6359)
  circle A0 centre (13, -9) radius 2
extrude "Extrude8" add sketch "Sketch9" along normal blind 10 contours A0 bodies 3
sketch "Sketch10" plane through (0, 0, 51.5) normal (0, 0, 1) x (-1, 0, 0)
  circle A0 centre (13, -9) radius 2
  circle A1 centre (13, -9) radius 1.6313
  constraint concentric A0 A1
sketch "Sketch11" plane through (0, 0, 0) normal (0, 1, 0) x (1, 0, 0)
  spline S0 degree 5 poles (-13, -51.5, 9) (-12.7384, -52.4143, 9) (-12.2618, -54.2148, 9) (-11.6869, -56.8319, 9) (-11.2049, -60.151, 9) (-11.1095, -63.9962, 9) (-11.5686, -67.5096, 9) (-12.6308, -70.6618, 9) (-14.3287, -73.4335, 9) (-16.6452, -75.8348, 9) (-19.5371, -77.8916, 9) (-22.2748, -79.2831, 9) (-24.5518, -80.1928, 9) (-26.1676, -80.7407, 9) (-27, -81, 9) knots 0 0 0 0 0 0 0.1 0.2 0.3 0.4 0.5 0.6 0.7 0.8 0.9 1 1 1 1 1 1
  point P0 (-13, -71)
sweep "Sweep1" add profiles "Sketch10" path "Sketch11" along S0 section 1 contours A1 bodies 3
move_body "Move1" bodies 3 to x (1, 0, 0) y (0, 1, 0) z (0, 0, 1) at (0, -64, 0)
